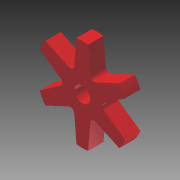
# Autodesk Inventor part: rubber intake star
Saved by Autodesk Inventor 2012 (Build 160160000, 160)
## iProperties
Created: 2013-07-07
Part Number: rubber intake star
Material: Default
Document SubType Name: Modeling
Designer: Bryce
Density: 1 g/cm^3
Author: Bryce
Autodesk Inventor part; units mm, degrees
ref_plane "YZ Plane" through (0, 0, 0) normal (1, 0, 0) x (0, 1, 0)
ref_plane "XZ Plane" through (0, 0, 0) normal (0, 1, 0) x (-1, 0, 0)
ref_plane "XY Plane" through (0, 0, 0) normal (0, 0, 1) x (1, 0, 0)
sketch "Sketch1" plane through (0, 0, 0) normal (0, 0, 1) x (1, 0, 0)
  arc A0 (4.7625, 37.8012) -> (-4.7625, 37.8012) centre (0, 0) ccw
  line L0 (-4.7625, 37.8012) -> (-7.0078, 12.1378)
  line L1 (0, 38.1) -> (0, 0) construction
  arc A1 (-4.7625, 37.8012) -> (-30.3555, 23.025) centre (0, 0) ccw construction
  line L2 (-7.0078, 12.1378) -> (7.0078, 12.1378) construction
  line L3 (7.0078, 12.1378) -> (14.0155, 0) construction
  line L4 (14.0155, 0) -> (7.0078, -12.1378) construction
  line L5 (7.0078, -12.1378) -> (-7.0078, -12.1378) construction
  line L6 (-7.0078, -12.1378) -> (-14.0155, 0) construction
  line L7 (-14.0155, 0) -> (-7.0078, 12.1378) construction
  line L8 (4.7625, 37.8012) -> (7.0078, 12.1378)
  line L9 (0, 0) -> (-32.9956, 19.05) construction
  line L10 (0, 0) -> (32.9956, 19.05) construction
  line L11 (0, 0) -> (-32.9956, -19.05) construction
  line L12 (0, 0) -> (32.9956, -19.05) construction
  line L13 (0, 0) -> (0, -38.1) construction
  line L14 (7.0078, 12.1378) -> (30.3555, 23.025)
  line L15 (14.0155, 0) -> (35.118, 14.7761)
  line L16 (14.0155, 0) -> (35.118, -14.7761)
  line L17 (7.0078, -12.1378) -> (30.3555, -23.025)
  arc A2 (30.3555, 23.025) -> (4.7625, 37.8012) centre (0, 0) ccw construction
  arc A3 (35.118, 14.7761) -> (30.3555, 23.025) centre (0, 0) ccw
  arc A4 (35.118, -14.7761) -> (35.118, 14.7761) centre (0, 0) ccw construction
  arc A5 (30.3555, -23.025) -> (35.118, -14.7761) centre (0, 0) ccw
  line L18 (7.0078, -12.1378) -> (4.7625, -37.8012)
  line L19 (-7.0078, -12.1378) -> (-4.7625, -37.8012)
  line L20 (-7.0078, -12.1378) -> (-30.3555, -23.025)
  line L21 (-14.0155, 0) -> (-35.118, -14.7761)
  line L22 (-14.0155, 0) -> (-35.118, 14.7761)
  line L23 (-7.0078, 12.1378) -> (-30.3555, 23.025)
  arc A6 (-30.3555, 23.025) -> (-35.118, 14.7761) centre (0, 0) ccw
  arc A7 (-35.118, 14.7761) -> (-35.118, -14.7761) centre (0, 0) ccw construction
  arc A8 (-35.118, -14.7761) -> (-30.3555, -23.025) centre (0, 0) ccw
  arc A9 (-30.3555, -23.025) -> (-4.7625, -37.8012) centre (0, 0) ccw construction
  arc A10 (-4.7625, -37.8012) -> (4.7625, -37.8012) centre (0, 0) ccw
  arc A11 (4.7625, -37.8012) -> (30.3555, -23.025) centre (0, 0) ccw construction
  circle A12 centre (0, 0) radius 6.35
  dimension "d10" = 38.1
  dimension "d1" = 9.525
  dimension "d2" = 4.7625
  dimension "d3" = 5
  dimension "d5" = 5
  dimension "d6" = 5
  dimension "d7" = 5
  dimension "d8" = 5
  dimension "d9" = 5
  dimension "d13" = 12.7
  constraints: 48 end point, 47 point on circle, 10 centre point, 7 equal length, 3 coincident, 2 perpendicular, 1 collinear, 1 horizontal, 1 vertical, 49 other
  measures "d1" distance of L8.start L0.start
  measures "d2" horizontal distance of L1.start L0.start
  measures "d3" angle of L1 L0
  measures "d5" angle of L10 L14
  measures "d6" angle of L10 L15
  measures "d7" angle of L12 L16
  measures "d8" angle of L12 L17
  measures "d9" angle of L13 L19
  measures "d13" diameter of A12
extrude "Extrusion1" add sketch "Sketch1" along normal blind 12.7
fillet "Fillet1" radius 3.175 6 edges at (7.0078, 12.1378, 6.35) (-7.0078, 12.1378, 6.35) (-14.0155, 0, 6.35) (-7.0078, -12.1378, 6.35) (7.0078, -12.1378, 6.35) (14.0155, 0, 6.35)
equation "\"d2\" = 0.5 * d1"
equation "\"d5\" = d3"
equation "\"d6\" = d3"
equation "\"d8\" = d6"
equation "\"d9\" = d8"
body "Solid1"
